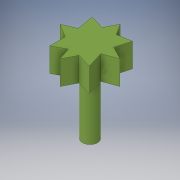
# Autodesk Inventor part: Wheels
Saved by Autodesk Inventor 2017 (Build 210142000, 142)
## iProperties
Created: 2020-01-18
Part Number: Wheels
Material: PBT Plastic
Document SubType Name: Modeling
Designer: Admin
Density: 1.31 g/cm^3
Appearance: Olive Green
Mass: 0.632861 g
Surface Area: 5.30312 cm^2
Volume: 0.4831 cm^3
Author: Admin
Autodesk Inventor part; units mm, degrees
ref_plane "YZ Plane" through (0, 0, 0) normal (1, 0, 0) x (0, 1, 0)
ref_plane "XZ Plane" through (0, 0, 0) normal (0, 1, 0) x (-1, 0, 0)
ref_plane "XY Plane" through (0, 0, 0) normal (0, 0, 1) x (1, 0, 0)
sketch "Sketch1" plane through (0, 0, 0) normal (0, 1, 0) x (-1, 0, 0)
  circle A0 centre (0, 0) radius 1.5875
  circle A1 centre (0, 0) radius 6.35
  dimension "d0" = 3.175
  dimension "d1" = 12.7
  constraints: 2 centre point, 2 coincident
  measures "d0" diameter of A0
  measures "d1" diameter of A1
extrude "Extrusion1" add sketch "Sketch1" along normal blind 5.08 contours A0 | A1
extrude "Extrusion2" add sketch "Sketch1" against normal blind 12.7 contours A0
sketch "Sketch2" plane through (0, 5.08, 0) normal (0, 1, 0) x (1, 0, 0)
  line L0 (6.3393, 0) -> (3.5604, 1.4472)
  line L1 (3.5604, 1.4472) -> (6.3393, 0)
  line L2 (6.3393, 0) -> (3.381, -1.08)
  line L3 (0, 0) -> (-1.7844, 0)
  circle A0 centre (0, 0) radius 6.35 projected
  line L4 (0, -6.35) -> (1.3494, -3.7028)
  line L5 (0, -6.35) -> (-0.8922, -3.6818)
  line L6 (-6.35, 0) -> (-3.4749, -1.7844)
  line L7 (-3.4749, -1.7844) -> (-6.35, 0)
  line L8 (-3.6501, 1.1418) -> (-6.35, 0)
  line L9 (0, 6.35) -> (1.509, 4.0476)
  line L10 (1.509, 4.0476) -> (0, 6.35)
  line L11 (0, 6.35) -> (-1.2759, 3.8681)
  line L12 (1.509, 4.0476) -> (4.4233, 4.556)
  line L13 (3.5604, 1.4472) -> (4.4233, 4.556)
  line L14 (3.381, -1.08) -> (4.4233, -4.556)
  line L15 (1.3494, -3.7028) -> (4.4233, -4.556)
  line L16 (-0.8922, -3.6818) -> (-3.4749, -5.0301)
  line L17 (-3.4749, -5.0301) -> (-3.4749, -1.7844)
  line L18 (-3.6501, 1.1418) -> (-4.2707, 4.6993)
  line L19 (-1.2759, 3.8681) -> (-4.2707, 4.6993)
  circle A1 centre (0, 0) radius 6.35
  constraints: 40 end point, 6 point on circle, 3 collinear, 2 perpendicular, 1 centre point, 1 coincident, 1 concentric, 1 horizontal, 1 parallel, 1 vertical
extrude "Extrusion3" cut sketch "Sketch2" against normal blind 5.08 contours L0 L13 A0 L14 L2 | L12 L9 A0 | A0 L4 L15 | L11 L19 A0 | A0 L6 L17 L16 L5 | L18 L8 A0
body "Solid1"
